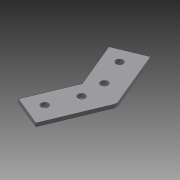
# Autodesk Inventor part: CornerBracketSheetMetal
Saved by Autodesk Inventor 2015 SP1 (Build 190203100, 203)
## iProperties
Created: 2015-02-01
Part Number: CornerBracketSheetMetal
Material: Generic
Document SubType Name: Sheet Metal
Designer: Andrew
Density: 1 g/cm^3
Sheet Metal Rule: Default
Appearance: Default
Author: Andrew
Autodesk Inventor part; units mm, degrees
ref_plane "YZ Plane" through (0, 0, 0) normal (1, 0, 0) x (0, 1, 0)
ref_plane "XZ Plane" through (0, 0, 0) normal (0, 1, 0) x (-1, 0, 0)
ref_plane "XY Plane" through (0, 0, 0) normal (0, 0, 1) x (1, 0, 0)
sketch "Sketch1" plane through (0, 0, 0) normal (0, 1, 0) x (-1, 0, 0)
  line L0 (0, 0) -> (21.3844, -51.6264)
  line L1 (21.3844, -51.6264) -> (47.9015, -40.6426)
  line L2 (47.9015, -40.6426) -> (31.0668, 0)
  line L3 (31.0668, 0) -> (47.9015, 40.6426)
  line L4 (47.9015, 40.6426) -> (21.3844, 51.6264)
  line L5 (21.3844, 51.6264) -> (0, 0)
  line L6 (31.0668, 0) -> (0, 0) construction
  line L7 (17.3204, 0) -> (56.2011, 93.8662) construction
  circle A0 centre (50.7089, 80.6068) radius 3.175
  circle A1 centre (40.9887, 57.1403) radius 3.175
  circle A2 centre (31.2686, 33.6737) radius 3.175
  circle A3 centre (21.5484, 10.2072) radius 3.175
  line L8 (13.0041, 3.7198) -> (13.0041, -3.7198) construction
  line L9 (13.0041, 0) -> (1.9044, 4.5976) construction
  line L10 (32.6076, 3.7198) -> (1.5408, 3.7198) construction
  line L11 (1.5408, -3.7198) -> (32.6076, -3.7198) construction
  circle A4 centre (21.5484, -10.2072) radius 3.175
  circle A5 centre (31.2686, -33.6737) radius 3.175
  dimension "d0" = 28.702
  dimension "d1" = 135
  dimension "d2" = 55.88
  dimension "d3" = 101.6
  dimension "d4" = 6.35
  dimension "d7" = 25.4
  dimension "d12" = 3.7198
  dimension "d13" = 12.7
  dimension "d14" = 12.0142
  dimension "d15" = 12.7
  measures "d0" distance of L0.end L1.end
  measures "d1" angle of L3 L2
  measures "d2" distance of L0.start L0.end
  measures "d3" distance of L7.start L7.end
  measures "d4" diameter of A0
  measures "d7" distance of A0.centre A1.centre
  measures "d12" distance between parallel lines of L6 L10
  measures "d13" distance from line of L9 A3.centre
  measures "d14" distance of L9.start L9.end
  measures "d15" distance between parallel lines of L7 L3
extrude "Plate1" add sketch "Sketch1" along normal blind 3.048 contours L5 L4 L3 L2 L1 L0
fillet "Corner Round1" radius 6.35 1 edges at (0, 1.524, 0)
equation "\"d3\" = 0.5 * CornerLength"
equation "\"BendRadius\" = Thickness"
equation "\"BendReliefWidth\" = Thickness"
equation "\"BendReliefDepth\" = 0.5 * Thickness"
equation "\"CornerReliefSize\" = 4 * Thickness"
equation "\"MinimumRemnant\" = 2 * Thickness"
equation "\"TransitionRadius\" = BendRadius"
equation "\"JacobiRadiusSize\" = BendRadius"
equation "\"GapSize\" = Thickness"
equation "\"d16\" = BendRadius"
equation "\"CornerLength\" = 203.2"
equation "\"Thickness\" = 3.048"
body "Solid1"
